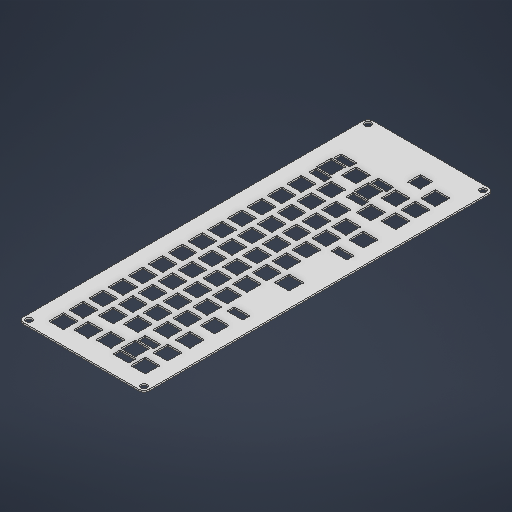
# Autodesk Inventor part: Top_Plate_Mkey
Saved by Autodesk Inventor 2026 (Build 300175050, 175E)
## iProperties
Created: 2025-06-24
Part Number: Top_Plate_Mkey
Material: Generic
Document SubType Name: Modeling
Designer: SaiAn
Density: 1 g/cm^3
Appearance: Default
Author: SaiAn
Autodesk Inventor part; units mm, degrees
ref_plane "YZ Plane" through (0, 0, 0) normal (1, 0, 0) x (0, 1, 0)
ref_plane "XZ Plane" through (0, 0, 0) normal (0, 1, 0) x (-1, 0, 0)
ref_plane "XY Plane" through (0, 0, 0) normal (0, 0, 1) x (1, 0, 0)
sketch "Sketch1" plane through (0, 0, 0) normal (0, 1, 0) x (-1, 0, 0)
  line L0 (0, 0) -> (120.47, 0)
  line L1 (120.47, 0) -> (120.47, -335.78)
  line L2 (120.47, -335.78) -> (0, -335.78)
  line L3 (104.715, -13.9387) -> (104.715, -26.9387)
  line L4 (90.715, -13.9387) -> (90.715, -26.9387)
  line L5 (104.215, -13.4387) -> (91.215, -13.4387)
  line L6 (104.215, -27.4387) -> (91.215, -27.4387)
  arc A0 (104.715, -13.9387) -> (104.215, -13.4387) centre (104.215, -13.9387) ccw
  arc A1 (104.215, -27.4387) -> (104.715, -26.9387) centre (104.215, -26.9387) ccw
  arc A2 (91.215, -13.4387) -> (90.715, -13.9387) centre (91.215, -13.9387) ccw
  arc A3 (90.715, -26.9387) -> (91.215, -27.4387) centre (91.215, -26.9387) ccw
  line L7 (104.715, -32.9887) -> (104.715, -45.9887)
  line L8 (90.715, -32.9887) -> (90.715, -45.9887)
  line L9 (104.215, -32.4887) -> (91.215, -32.4887)
  line L10 (104.215, -46.4887) -> (91.215, -46.4887)
  arc A4 (104.715, -32.9887) -> (104.215, -32.4887) centre (104.215, -32.9887) ccw
  arc A5 (104.215, -46.4887) -> (104.715, -45.9887) centre (104.215, -45.9887) ccw
  arc A6 (91.215, -32.4887) -> (90.715, -32.9887) centre (91.215, -32.9887) ccw
  arc A7 (90.715, -45.9887) -> (91.215, -46.4887) centre (91.215, -45.9887) ccw
  line L11 (104.715, -52.0387) -> (104.715, -65.0387)
  line L12 (90.715, -52.0387) -> (90.715, -65.0387)
  line L13 (104.215, -51.5387) -> (91.215, -51.5387)
  line L14 (104.215, -65.5387) -> (91.215, -65.5387)
  arc A8 (104.715, -52.0387) -> (104.215, -51.5387) centre (104.215, -52.0387) ccw
  arc A9 (104.215, -65.5387) -> (104.715, -65.0387) centre (104.215, -65.0387) ccw
  arc A10 (91.215, -51.5387) -> (90.715, -52.0387) centre (91.215, -52.0387) ccw
  arc A11 (90.715, -65.0387) -> (91.215, -65.5387) centre (91.215, -65.0387) ccw
  line L15 (104.715, -71.0887) -> (104.715, -84.0887)
  line L16 (90.715, -71.0887) -> (90.715, -84.0887)
  line L17 (104.215, -70.5887) -> (91.215, -70.5887)
  line L18 (104.215, -84.5887) -> (91.215, -84.5887)
  arc A12 (104.715, -71.0887) -> (104.215, -70.5887) centre (104.215, -71.0887) ccw
  arc A13 (104.215, -84.5887) -> (104.715, -84.0887) centre (104.215, -84.0887) ccw
  arc A14 (91.215, -70.5887) -> (90.715, -71.0887) centre (91.215, -71.0887) ccw
  arc A15 (90.715, -84.0887) -> (91.215, -84.5887) centre (91.215, -84.0887) ccw
  line L19 (104.715, -90.1387) -> (104.715, -103.1387)
  line L20 (90.715, -90.1387) -> (90.715, -103.1387)
  line L21 (104.215, -89.6387) -> (91.215, -89.6387)
  line L22 (104.215, -103.6387) -> (91.215, -103.6387)
  arc A16 (104.715, -90.1387) -> (104.215, -89.6387) centre (104.215, -90.1387) ccw
  arc A17 (104.215, -103.6387) -> (104.715, -103.1387) centre (104.215, -103.1387) ccw
  arc A18 (91.215, -89.6387) -> (90.715, -90.1387) centre (91.215, -90.1387) ccw
  arc A19 (90.715, -103.1387) -> (91.215, -103.6387) centre (91.215, -103.1387) ccw
  line L23 (104.715, -109.1887) -> (104.715, -122.1887)
  line L24 (90.715, -109.1887) -> (90.715, -122.1887)
  line L25 (104.215, -108.6887) -> (91.215, -108.6887)
  line L26 (104.215, -122.6887) -> (91.215, -122.6887)
  arc A20 (104.715, -109.1887) -> (104.215, -108.6887) centre (104.215, -109.1887) ccw
  arc A21 (104.215, -122.6887) -> (104.715, -122.1887) centre (104.215, -122.1887) ccw
  arc A22 (91.215, -108.6887) -> (90.715, -109.1887) centre (91.215, -109.1887) ccw
  arc A23 (90.715, -122.1887) -> (91.215, -122.6887) centre (91.215, -122.1887) ccw
  line L27 (104.715, -128.2387) -> (104.715, -141.2387)
  line L28 (90.715, -128.2387) -> (90.715, -141.2387)
  line L29 (104.215, -127.7387) -> (91.215, -127.7387)
  line L30 (104.215, -141.7387) -> (91.215, -141.7387)
  arc A24 (104.715, -128.2387) -> (104.215, -127.7387) centre (104.215, -128.2387) ccw
  arc A25 (104.215, -141.7387) -> (104.715, -141.2387) centre (104.215, -141.2387) ccw
  arc A26 (91.215, -127.7387) -> (90.715, -128.2387) centre (91.215, -128.2387) ccw
  arc A27 (90.715, -141.2387) -> (91.215, -141.7387) centre (91.215, -141.2387) ccw
  line L31 (104.715, -147.2887) -> (104.715, -160.2887)
  line L32 (90.715, -147.2887) -> (90.715, -160.2887)
  line L33 (104.215, -146.7887) -> (91.215, -146.7887)
  line L34 (104.215, -160.7887) -> (91.215, -160.7887)
  arc A28 (104.715, -147.2887) -> (104.215, -146.7887) centre (104.215, -147.2887) ccw
  arc A29 (104.215, -160.7887) -> (104.715, -160.2887) centre (104.215, -160.2887) ccw
  arc A30 (91.215, -146.7887) -> (90.715, -147.2887) centre (91.215, -147.2887) ccw
  arc A31 (90.715, -160.2887) -> (91.215, -160.7887) centre (91.215, -160.2887) ccw
  line L35 (104.715, -166.3387) -> (104.715, -179.3387)
  line L36 (90.715, -166.3387) -> (90.715, -179.3387)
  line L37 (104.215, -165.8387) -> (91.215, -165.8387)
  line L38 (104.215, -179.8387) -> (91.215, -179.8387)
  arc A32 (104.715, -166.3387) -> (104.215, -165.8387) centre (104.215, -166.3387) ccw
  arc A33 (104.215, -179.8387) -> (104.715, -179.3387) centre (104.215, -179.3387) ccw
  arc A34 (91.215, -165.8387) -> (90.715, -166.3387) centre (91.215, -166.3387) ccw
  arc A35 (90.715, -179.3387) -> (91.215, -179.8387) centre (91.215, -179.3387) ccw
  line L39 (104.715, -185.3887) -> (104.715, -198.3887)
  line L40 (90.715, -185.3887) -> (90.715, -198.3887)
  line L41 (104.215, -184.8887) -> (91.215, -184.8887)
  line L42 (104.215, -198.8887) -> (91.215, -198.8887)
  arc A36 (104.715, -185.3887) -> (104.215, -184.8887) centre (104.215, -185.3887) ccw
  arc A37 (104.215, -198.8887) -> (104.715, -198.3887) centre (104.215, -198.3887) ccw
  arc A38 (91.215, -184.8887) -> (90.715, -185.3887) centre (91.215, -185.3887) ccw
  arc A39 (90.715, -198.3887) -> (91.215, -198.8887) centre (91.215, -198.3887) ccw
  line L43 (104.715, -204.4387) -> (104.715, -217.4387)
  line L44 (90.715, -204.4387) -> (90.715, -217.4387)
  line L45 (104.215, -203.9387) -> (91.215, -203.9387)
  line L46 (104.215, -217.9387) -> (91.215, -217.9387)
  arc A40 (104.715, -204.4387) -> (104.215, -203.9387) centre (104.215, -204.4387) ccw
  arc A41 (104.215, -217.9387) -> (104.715, -217.4387) centre (104.215, -217.4387) ccw
  arc A42 (91.215, -203.9387) -> (90.715, -204.4387) centre (91.215, -204.4387) ccw
  arc A43 (90.715, -217.4387) -> (91.215, -217.9387) centre (91.215, -217.4387) ccw
  line L47 (104.715, -223.4887) -> (104.715, -236.4887)
  line L48 (90.715, -223.4887) -> (90.715, -236.4887)
  line L49 (104.215, -222.9887) -> (91.215, -222.9887)
  line L50 (104.215, -236.9887) -> (91.215, -236.9887)
  arc A44 (104.715, -223.4887) -> (104.215, -222.9887) centre (104.215, -223.4887) ccw
  arc A45 (104.215, -236.9887) -> (104.715, -236.4887) centre (104.215, -236.4887) ccw
  arc A46 (91.215, -222.9887) -> (90.715, -223.4887) centre (91.215, -223.4887) ccw
  arc A47 (90.715, -236.4887) -> (91.215, -236.9887) centre (91.215, -236.4887) ccw
  line L51 (104.715, -242.5387) -> (104.715, -255.5387)
  line L52 (90.715, -242.5387) -> (90.715, -255.5387)
  line L53 (104.215, -242.0387) -> (91.215, -242.0387)
  line L54 (104.215, -256.0387) -> (91.215, -256.0387)
  arc A48 (104.715, -242.5387) -> (104.215, -242.0387) centre (104.215, -242.5387) ccw
  arc A49 (104.215, -256.0387) -> (104.715, -255.5387) centre (104.215, -255.5387) ccw
  arc A50 (91.215, -242.0387) -> (90.715, -242.5387) centre (91.215, -242.5387) ccw
  arc A51 (90.715, -255.5387) -> (91.215, -256.0387) centre (91.215, -255.5387) ccw
  line L55 (104.715, -271.1137) -> (104.715, -284.1137)
  line L56 (90.715, -271.1137) -> (90.715, -284.1137)
  line L57 (104.215, -270.6137) -> (91.215, -270.6137)
  line L58 (104.215, -284.6137) -> (91.215, -284.6137)
  arc A52 (104.715, -271.1137) -> (104.215, -270.6137) centre (104.215, -271.1137) ccw
  arc A53 (104.215, -284.6137) -> (104.715, -284.1137) centre (104.215, -284.1137) ccw
  arc A54 (91.215, -270.6137) -> (90.715, -271.1137) centre (91.215, -271.1137) ccw
  arc A55 (90.715, -284.1137) -> (91.215, -284.6137) centre (91.215, -284.1137) ccw
  line L59 (103.715, -262.6757) -> (103.715, -268.6757)
  line L60 (88.715, -262.6757) -> (88.715, -268.6757)
  line L61 (103.215, -262.1757) -> (89.215, -262.1757)
  line L62 (103.215, -269.1757) -> (89.215, -269.1757)
  arc A56 (103.715, -262.6757) -> (103.215, -262.1757) centre (103.215, -262.6757) ccw
  arc A57 (103.215, -269.1757) -> (103.715, -268.6757) centre (103.215, -268.6757) ccw
  arc A58 (89.215, -262.1757) -> (88.715, -262.6757) centre (89.215, -262.6757) ccw
  arc A59 (88.715, -268.6757) -> (89.215, -269.1757) centre (89.215, -268.6757) ccw
  line L63 (103.715, -286.5517) -> (103.715, -292.5517)
  line L64 (88.715, -286.5517) -> (88.715, -292.5517)
  line L65 (103.215, -286.0517) -> (89.215, -286.0517)
  line L66 (103.215, -293.0517) -> (89.215, -293.0517)
  arc A60 (103.715, -286.5517) -> (103.215, -286.0517) centre (103.215, -286.5517) ccw
  arc A61 (103.215, -293.0517) -> (103.715, -292.5517) centre (103.215, -292.5517) ccw
  arc A62 (89.215, -286.0517) -> (88.715, -286.5517) centre (89.215, -286.5517) ccw
  arc A63 (88.715, -292.5517) -> (89.215, -293.0517) centre (89.215, -292.5517) ccw
  line L67 (85.665, -18.7012) -> (85.665, -31.7012)
  line L68 (71.665, -18.7012) -> (71.665, -31.7012)
  line L69 (85.165, -18.2012) -> (72.165, -18.2012)
  line L70 (85.165, -32.2012) -> (72.165, -32.2012)
  arc A64 (85.665, -18.7012) -> (85.165, -18.2012) centre (85.165, -18.7012) ccw
  arc A65 (85.165, -32.2012) -> (85.665, -31.7012) centre (85.165, -31.7012) ccw
  arc A66 (72.165, -18.2012) -> (71.665, -18.7012) centre (72.165, -18.7012) ccw
  arc A67 (71.665, -31.7012) -> (72.165, -32.2012) centre (72.165, -31.7012) ccw
  line L71 (85.665, -42.5137) -> (85.665, -55.5137)
  line L72 (71.665, -42.5137) -> (71.665, -55.5137)
  line L73 (85.165, -42.0137) -> (72.165, -42.0137)
  line L74 (85.165, -56.0137) -> (72.165, -56.0137)
  arc A68 (85.665, -42.5137) -> (85.165, -42.0137) centre (85.165, -42.5137) ccw
  arc A69 (85.165, -56.0137) -> (85.665, -55.5137) centre (85.165, -55.5137) ccw
  arc A70 (72.165, -42.0137) -> (71.665, -42.5137) centre (72.165, -42.5137) ccw
  arc A71 (71.665, -55.5137) -> (72.165, -56.0137) centre (72.165, -55.5137) ccw
  line L75 (85.665, -61.5637) -> (85.665, -74.5637)
  line L76 (71.665, -61.5637) -> (71.665, -74.5637)
  line L77 (85.165, -61.0637) -> (72.165, -61.0637)
  line L78 (85.165, -75.0637) -> (72.165, -75.0637)
  arc A72 (85.665, -61.5637) -> (85.165, -61.0637) centre (85.165, -61.5637) ccw
  arc A73 (85.165, -75.0637) -> (85.665, -74.5637) centre (85.165, -74.5637) ccw
  arc A74 (72.165, -61.0637) -> (71.665, -61.5637) centre (72.165, -61.5637) ccw
  arc A75 (71.665, -74.5637) -> (72.165, -75.0637) centre (72.165, -74.5637) ccw
  line L79 (85.665, -80.6137) -> (85.665, -93.6137)
  line L80 (71.665, -80.6137) -> (71.665, -93.6137)
  line L81 (85.165, -80.1137) -> (72.165, -80.1137)
  line L82 (85.165, -94.1137) -> (72.165, -94.1137)
  arc A76 (85.665, -80.6137) -> (85.165, -80.1137) centre (85.165, -80.6137) ccw
  arc A77 (85.165, -94.1137) -> (85.665, -93.6137) centre (85.165, -93.6137) ccw
  arc A78 (72.165, -80.1137) -> (71.665, -80.6137) centre (72.165, -80.6137) ccw
  arc A79 (71.665, -93.6137) -> (72.165, -94.1137) centre (72.165, -93.6137) ccw
  line L83 (85.665, -99.6637) -> (85.665, -112.6637)
  line L84 (71.665, -99.6637) -> (71.665, -112.6637)
  line L85 (85.165, -99.1637) -> (72.165, -99.1637)
  line L86 (85.165, -113.1637) -> (72.165, -113.1637)
  arc A80 (85.665, -99.6637) -> (85.165, -99.1637) centre (85.165, -99.6637) ccw
  arc A81 (85.165, -113.1637) -> (85.665, -112.6637) centre (85.165, -112.6637) ccw
  arc A82 (72.165, -99.1637) -> (71.665, -99.6637) centre (72.165, -99.6637) ccw
  arc A83 (71.665, -112.6637) -> (72.165, -113.1637) centre (72.165, -112.6637) ccw
  line L87 (85.665, -118.7137) -> (85.665, -131.7137)
  line L88 (71.665, -118.7137) -> (71.665, -131.7137)
  line L89 (85.165, -118.2137) -> (72.165, -118.2137)
  line L90 (85.165, -132.2137) -> (72.165, -132.2137)
  arc A84 (85.665, -118.7137) -> (85.165, -118.2137) centre (85.165, -118.7137) ccw
  arc A85 (85.165, -132.2137) -> (85.665, -131.7137) centre (85.165, -131.7137) ccw
  arc A86 (72.165, -118.2137) -> (71.665, -118.7137) centre (72.165, -118.7137) ccw
  arc A87 (71.665, -131.7137) -> (72.165, -132.2137) centre (72.165, -131.7137) ccw
  line L91 (85.665, -137.7637) -> (85.665, -150.7637)
  line L92 (71.665, -137.7637) -> (71.665, -150.7637)
  line L93 (85.165, -137.2637) -> (72.165, -137.2637)
  line L94 (85.165, -151.2637) -> (72.165, -151.2637)
  arc A88 (85.665, -137.7637) -> (85.165, -137.2637) centre (85.165, -137.7637) ccw
  arc A89 (85.165, -151.2637) -> (85.665, -150.7637) centre (85.165, -150.7637) ccw
  arc A90 (72.165, -137.2637) -> (71.665, -137.7637) centre (72.165, -137.7637) ccw
  arc A91 (71.665, -150.7637) -> (72.165, -151.2637) centre (72.165, -150.7637) ccw
  line L95 (85.665, -156.8137) -> (85.665, -169.8137)
  line L96 (71.665, -156.8137) -> (71.665, -169.8137)
  line L97 (85.165, -156.3137) -> (72.165, -156.3137)
  line L98 (85.165, -170.3137) -> (72.165, -170.3137)
  arc A92 (85.665, -156.8137) -> (85.165, -156.3137) centre (85.165, -156.8137) ccw
  arc A93 (85.165, -170.3137) -> (85.665, -169.8137) centre (85.165, -169.8137) ccw
  arc A94 (72.165, -156.3137) -> (71.665, -156.8137) centre (72.165, -156.8137) ccw
  arc A95 (71.665, -169.8137) -> (72.165, -170.3137) centre (72.165, -169.8137) ccw
  line L99 (85.665, -175.8637) -> (85.665, -188.8637)
  line L100 (71.665, -175.8637) -> (71.665, -188.8637)
  line L101 (85.165, -175.3637) -> (72.165, -175.3637)
  line L102 (85.165, -189.3637) -> (72.165, -189.3637)
  arc A96 (85.665, -175.8637) -> (85.165, -175.3637) centre (85.165, -175.8637) ccw
  arc A97 (85.165, -189.3637) -> (85.665, -188.8637) centre (85.165, -188.8637) ccw
  arc A98 (72.165, -175.3637) -> (71.665, -175.8637) centre (72.165, -175.8637) ccw
  arc A99 (71.665, -188.8637) -> (72.165, -189.3637) centre (72.165, -188.8637) ccw
  line L103 (85.665, -194.9137) -> (85.665, -207.9137)
  line L104 (71.665, -194.9137) -> (71.665, -207.9137)
  line L105 (85.165, -194.4137) -> (72.165, -194.4137)
  line L106 (85.165, -208.4137) -> (72.165, -208.4137)
  arc A100 (85.665, -194.9137) -> (85.165, -194.4137) centre (85.165, -194.9137) ccw
  arc A101 (85.165, -208.4137) -> (85.665, -207.9137) centre (85.165, -207.9137) ccw
  arc A102 (72.165, -194.4137) -> (71.665, -194.9137) centre (72.165, -194.9137) ccw
  arc A103 (71.665, -207.9137) -> (72.165, -208.4137) centre (72.165, -207.9137) ccw
  line L107 (85.665, -213.9637) -> (85.665, -226.9637)
  line L108 (71.665, -213.9637) -> (71.665, -226.9637)
  line L109 (85.165, -213.4637) -> (72.165, -213.4637)
  line L110 (85.165, -227.4637) -> (72.165, -227.4637)
  arc A104 (85.665, -213.9637) -> (85.165, -213.4637) centre (85.165, -213.9637) ccw
  arc A105 (85.165, -227.4637) -> (85.665, -226.9637) centre (85.165, -226.9637) ccw
  arc A106 (72.165, -213.4637) -> (71.665, -213.9637) centre (72.165, -213.9637) ccw
  arc A107 (71.665, -226.9637) -> (72.165, -227.4637) centre (72.165, -226.9637) ccw
  line L111 (85.665, -233.0137) -> (85.665, -246.0137)
  line L112 (71.665, -233.0137) -> (71.665, -246.0137)
  line L113 (85.165, -232.5137) -> (72.165, -232.5137)
  line L114 (85.165, -246.5137) -> (72.165, -246.5137)
  arc A108 (85.665, -233.0137) -> (85.165, -232.5137) centre (85.165, -233.0137) ccw
  arc A109 (85.165, -246.5137) -> (85.665, -246.0137) centre (85.165, -246.0137) ccw
  arc A110 (72.165, -232.5137) -> (71.665, -233.0137) centre (72.165, -233.0137) ccw
  arc A111 (71.665, -246.0137) -> (72.165, -246.5137) centre (72.165, -246.0137) ccw
  line L115 (85.665, -252.0637) -> (85.665, -265.0637)
  line L116 (71.665, -252.0637) -> (71.665, -265.0637)
  line L117 (85.165, -251.5637) -> (72.165, -251.5637)
  line L118 (85.165, -265.5637) -> (72.165, -265.5637)
  arc A112 (85.665, -252.0637) -> (85.165, -251.5637) centre (85.165, -252.0637) ccw
  arc A113 (85.165, -265.5637) -> (85.665, -265.0637) centre (85.165, -265.0637) ccw
  arc A114 (72.165, -251.5637) -> (71.665, -252.0637) centre (72.165, -252.0637) ccw
  arc A115 (71.665, -265.0637) -> (72.165, -265.5637) centre (72.165, -265.0637) ccw
  line L119 (85.665, -275.8762) -> (85.665, -288.8762)
  line L120 (71.665, -275.8762) -> (71.665, -288.8762)
  line L121 (85.165, -275.3762) -> (72.165, -275.3762)
  line L122 (85.165, -289.3762) -> (72.165, -289.3762)
  arc A116 (85.665, -275.8762) -> (85.165, -275.3762) centre (85.165, -275.8762) ccw
  arc A117 (85.165, -289.3762) -> (85.665, -288.8762) centre (85.165, -288.8762) ccw
  arc A118 (72.165, -275.3762) -> (71.665, -275.8762) centre (72.165, -275.8762) ccw
  arc A119 (71.665, -288.8762) -> (72.165, -289.3762) centre (72.165, -288.8762) ccw
  line L123 (66.615, -21.0825) -> (66.615, -34.0825)
  line L124 (52.615, -21.0825) -> (52.615, -34.0825)
  line L125 (66.115, -20.5825) -> (53.115, -20.5825)
  line L126 (66.115, -34.5825) -> (53.115, -34.5825)
  arc A120 (66.615, -21.0825) -> (66.115, -20.5825) centre (66.115, -21.0825) ccw
  arc A121 (66.115, -34.5825) -> (66.615, -34.0825) centre (66.115, -34.0825) ccw
  arc A122 (53.115, -20.5825) -> (52.615, -21.0825) centre (53.115, -21.0825) ccw
  arc A123 (52.615, -34.0825) -> (53.115, -34.5825) centre (53.115, -34.0825) ccw
  line L127 (66.615, -47.2762) -> (66.615, -60.2762)
  line L128 (52.615, -47.2762) -> (52.615, -60.2762)
  line L129 (66.115, -46.7762) -> (53.115, -46.7762)
  line L130 (66.115, -60.7762) -> (53.115, -60.7762)
  arc A124 (66.615, -47.2762) -> (66.115, -46.7762) centre (66.115, -47.2762) ccw
  arc A125 (66.115, -60.7762) -> (66.615, -60.2762) centre (66.115, -60.2762) ccw
  arc A126 (53.115, -46.7762) -> (52.615, -47.2762) centre (53.115, -47.2762) ccw
  arc A127 (52.615, -60.2762) -> (53.115, -60.7762) centre (53.115, -60.2762) ccw
  line L131 (66.615, -66.3262) -> (66.615, -79.3262)
  line L132 (52.615, -66.3262) -> (52.615, -79.3262)
  line L133 (66.115, -65.8262) -> (53.115, -65.8262)
  line L134 (66.115, -79.8262) -> (53.115, -79.8262)
  arc A128 (66.615, -66.3262) -> (66.115, -65.8262) centre (66.115, -66.3262) ccw
  arc A129 (66.115, -79.8262) -> (66.615, -79.3262) centre (66.115, -79.3262) ccw
  arc A130 (53.115, -65.8262) -> (52.615, -66.3262) centre (53.115, -66.3262) ccw
  arc A131 (52.615, -79.3262) -> (53.115, -79.8262) centre (53.115, -79.3262) ccw
  line L135 (66.615, -85.3762) -> (66.615, -98.3762)
  line L136 (52.615, -85.3762) -> (52.615, -98.3762)
  line L137 (66.115, -84.8762) -> (53.115, -84.8762)
  line L138 (66.115, -98.8762) -> (53.115, -98.8762)
  arc A132 (66.615, -85.3762) -> (66.115, -84.8762) centre (66.115, -85.3762) ccw
  arc A133 (66.115, -98.8762) -> (66.615, -98.3762) centre (66.115, -98.3762) ccw
  arc A134 (53.115, -84.8762) -> (52.615, -85.3762) centre (53.115, -85.3762) ccw
  arc A135 (52.615, -98.3762) -> (53.115, -98.8762) centre (53.115, -98.3762) ccw
  line L139 (66.615, -104.4262) -> (66.615, -117.4262)
  line L140 (52.615, -104.4262) -> (52.615, -117.4262)
  line L141 (66.115, -103.9262) -> (53.115, -103.9262)
  line L142 (66.115, -117.9262) -> (53.115, -117.9262)
  arc A136 (66.615, -104.4262) -> (66.115, -103.9262) centre (66.115, -104.4262) ccw
  arc A137 (66.115, -117.9262) -> (66.615, -117.4262) centre (66.115, -117.4262) ccw
  arc A138 (53.115, -103.9262) -> (52.615, -104.4262) centre (53.115, -104.4262) ccw
  arc A139 (52.615, -117.4262) -> (53.115, -117.9262) centre (53.115, -117.4262) ccw
  line L143 (66.615, -123.4762) -> (66.615, -136.4762)
  line L144 (52.615, -123.4762) -> (52.615, -136.4762)
  line L145 (66.115, -122.9762) -> (53.115, -122.9762)
  line L146 (66.115, -136.9762) -> (53.115, -136.9762)
  arc A140 (66.615, -123.4762) -> (66.115, -122.9762) centre (66.115, -123.4762) ccw
  arc A141 (66.115, -136.9762) -> (66.615, -136.4762) centre (66.115, -136.4762) ccw
  arc A142 (53.115, -122.9762) -> (52.615, -123.4762) centre (53.115, -123.4762) ccw
  arc A143 (52.615, -136.4762) -> (53.115, -136.9762) centre (53.115, -136.4762) ccw
  line L147 (66.615, -142.5262) -> (66.615, -155.5262)
  line L148 (52.615, -142.5262) -> (52.615, -155.5262)
  line L149 (66.115, -142.0262) -> (53.115, -142.0262)
  line L150 (66.115, -156.0262) -> (53.115, -156.0262)
  arc A144 (66.615, -142.5262) -> (66.115, -142.0262) centre (66.115, -142.5262) ccw
  arc A145 (66.115, -156.0262) -> (66.615, -155.5262) centre (66.115, -155.5262) ccw
  arc A146 (53.115, -142.0262) -> (52.615, -142.5262) centre (53.115, -142.5262) ccw
  arc A147 (52.615, -155.5262) -> (53.115, -156.0262) centre (53.115, -155.5262) ccw
  line L151 (66.615, -161.5762) -> (66.615, -174.5762)
  line L152 (52.615, -161.5762) -> (52.615, -174.5762)
  line L153 (66.115, -161.0762) -> (53.115, -161.0762)
  line L154 (66.115, -175.0762) -> (53.115, -175.0762)
  arc A148 (66.615, -161.5762) -> (66.115, -161.0762) centre (66.115, -161.5762) ccw
  arc A149 (66.115, -175.0762) -> (66.615, -174.5762) centre (66.115, -174.5762) ccw
  arc A150 (53.115, -161.0762) -> (52.615, -161.5762) centre (53.115, -161.5762) ccw
  arc A151 (52.615, -174.5762) -> (53.115, -175.0762) centre (53.115, -174.5762) ccw
  line L155 (66.615, -180.6262) -> (66.615, -193.6262)
  line L156 (52.615, -180.6262) -> (52.615, -193.6262)
  line L157 (66.115, -180.1262) -> (53.115, -180.1262)
  line L158 (66.115, -194.1262) -> (53.115, -194.1262)
  arc A152 (66.615, -180.6262) -> (66.115, -180.1262) centre (66.115, -180.6262) ccw
  arc A153 (66.115, -194.1262) -> (66.615, -193.6262) centre (66.115, -193.6262) ccw
  arc A154 (53.115, -180.1262) -> (52.615, -180.6262) centre (53.115, -180.6262) ccw
  arc A155 (52.615, -193.6262) -> (53.115, -194.1262) centre (53.115, -193.6262) ccw
  line L159 (66.615, -199.6762) -> (66.615, -212.6762)
  line L160 (52.615, -199.6762) -> (52.615, -212.6762)
  line L161 (66.115, -199.1762) -> (53.115, -199.1762)
  line L162 (66.115, -213.1762) -> (53.115, -213.1762)
  arc A156 (66.615, -199.6762) -> (66.115, -199.1762) centre (66.115, -199.6762) ccw
  arc A157 (66.115, -213.1762) -> (66.615, -212.6762) centre (66.115, -212.6762) ccw
  arc A158 (53.115, -199.1762) -> (52.615, -199.6762) centre (53.115, -199.6762) ccw
  arc A159 (52.615, -212.6762) -> (53.115, -213.1762) centre (53.115, -212.6762) ccw
  line L163 (66.615, -218.7262) -> (66.615, -231.7262)
  line L164 (52.615, -218.7262) -> (52.615, -231.7262)
  line L165 (66.115, -218.2262) -> (53.115, -218.2262)
  line L166 (66.115, -232.2262) -> (53.115, -232.2262)
  arc A160 (66.615, -218.7262) -> (66.115, -218.2262) centre (66.115, -218.7262) ccw
  arc A161 (66.115, -232.2262) -> (66.615, -231.7262) centre (66.115, -231.7262) ccw
  arc A162 (53.115, -218.2262) -> (52.615, -218.7262) centre (53.115, -218.7262) ccw
  arc A163 (52.615, -231.7262) -> (53.115, -232.2262) centre (53.115, -231.7262) ccw
  line L167 (66.615, -237.7762) -> (66.615, -250.7762)
  line L168 (52.615, -237.7762) -> (52.615, -250.7762)
  line L169 (66.115, -237.2762) -> (53.115, -237.2762)
  line L170 (66.115, -251.2762) -> (53.115, -251.2762)
  arc A164 (66.615, -237.7762) -> (66.115, -237.2762) centre (66.115, -237.7762) ccw
  arc A165 (66.115, -251.2762) -> (66.615, -250.7762) centre (66.115, -250.7762) ccw
  arc A166 (53.115, -237.2762) -> (52.615, -237.7762) centre (53.115, -237.7762) ccw
  arc A167 (52.615, -250.7762) -> (53.115, -251.2762) centre (53.115, -250.7762) ccw
  line L171 (66.615, -268.7325) -> (66.615, -281.7325)
  line L172 (52.615, -268.7325) -> (52.615, -281.7325)
  line L173 (66.115, -268.2325) -> (53.115, -268.2325)
  line L174 (66.115, -282.2325) -> (53.115, -282.2325)
  arc A168 (66.615, -268.7325) -> (66.115, -268.2325) centre (66.115, -268.7325) ccw
  arc A169 (66.115, -282.2325) -> (66.615, -281.7325) centre (66.115, -281.7325) ccw
  arc A170 (53.115, -268.2325) -> (52.615, -268.7325) centre (53.115, -268.7325) ccw
  arc A171 (52.615, -281.7325) -> (53.115, -282.2325) centre (53.115, -281.7325) ccw
  line L175 (65.615, -260.2945) -> (65.615, -266.2945)
  line L176 (50.615, -260.2945) -> (50.615, -266.2945)
  line L177 (65.115, -259.7945) -> (51.115, -259.7945)
  line L178 (65.115, -266.7945) -> (51.115, -266.7945)
  arc A172 (65.615, -260.2945) -> (65.115, -259.7945) centre (65.115, -260.2945) ccw
  arc A173 (65.115, -266.7945) -> (65.615, -266.2945) centre (65.115, -266.2945) ccw
  arc A174 (51.115, -259.7945) -> (50.615, -260.2945) centre (51.115, -260.2945) ccw
  arc A175 (50.615, -266.2945) -> (51.115, -266.7945) centre (51.115, -266.2945) ccw
  line L179 (65.615, -284.1705) -> (65.615, -290.1705)
  line L180 (50.615, -284.1705) -> (50.615, -290.1705)
  line L181 (65.115, -283.6705) -> (51.115, -283.6705)
  line L182 (65.115, -290.6705) -> (51.115, -290.6705)
  arc A176 (65.615, -284.1705) -> (65.115, -283.6705) centre (65.115, -284.1705) ccw
  arc A177 (65.115, -290.6705) -> (65.615, -290.1705) centre (65.115, -290.1705) ccw
  arc A178 (51.115, -283.6705) -> (50.615, -284.1705) centre (51.115, -284.1705) ccw
  arc A179 (50.615, -290.1705) -> (51.115, -290.6705) centre (51.115, -290.1705) ccw
  line L183 (47.565, -25.845) -> (47.565, -38.845)
  line L184 (33.565, -25.845) -> (33.565, -38.845)
  line L185 (47.065, -25.345) -> (34.065, -25.345)
  line L186 (47.065, -39.345) -> (34.065, -39.345)
  arc A180 (47.565, -25.845) -> (47.065, -25.345) centre (47.065, -25.845) ccw
  arc A181 (47.065, -39.345) -> (47.565, -38.845) centre (47.065, -38.845) ccw
  arc A182 (34.065, -25.345) -> (33.565, -25.845) centre (34.065, -25.845) ccw
  arc A183 (33.565, -38.845) -> (34.065, -39.345) centre (34.065, -38.845) ccw
  line L187 (46.565, -17.407) -> (46.565, -23.407)
  line L188 (31.565, -17.407) -> (31.565, -23.407)
  line L189 (46.065, -16.907) -> (32.065, -16.907)
  line L190 (46.065, -23.907) -> (32.065, -23.907)
  arc A184 (46.565, -17.407) -> (46.065, -16.907) centre (46.065, -17.407) ccw
  arc A185 (46.065, -23.907) -> (46.565, -23.407) centre (46.065, -23.407) ccw
  arc A186 (32.065, -16.907) -> (31.565, -17.407) centre (32.065, -17.407) ccw
  arc A187 (31.565, -23.407) -> (32.065, -23.907) centre (32.065, -23.407) ccw
  line L191 (46.565, -41.283) -> (46.565, -47.283)
  line L192 (31.565, -41.283) -> (31.565, -47.283)
  line L193 (46.065, -40.783) -> (32.065, -40.783)
  line L194 (46.065, -47.783) -> (32.065, -47.783)
  arc A188 (46.565, -41.283) -> (46.065, -40.783) centre (46.065, -41.283) ccw
  arc A189 (46.065, -47.783) -> (46.565, -47.283) centre (46.065, -47.283) ccw
  arc A190 (32.065, -40.783) -> (31.565, -41.283) centre (32.065, -41.283) ccw
  arc A191 (31.565, -47.283) -> (32.065, -47.783) centre (32.065, -47.283) ccw
  line L195 (47.565, -56.8012) -> (47.565, -69.8012)
  line L196 (33.565, -56.8012) -> (33.565, -69.8012)
  line L197 (47.065, -56.3012) -> (34.065, -56.3012)
  line L198 (47.065, -70.3012) -> (34.065, -70.3012)
  arc A192 (47.565, -56.8012) -> (47.065, -56.3012) centre (47.065, -56.8012) ccw
  arc A193 (47.065, -70.3012) -> (47.565, -69.8012) centre (47.065, -69.8012) ccw
  arc A194 (34.065, -56.3012) -> (33.565, -56.8012) centre (34.065, -56.8012) ccw
  arc A195 (33.565, -69.8012) -> (34.065, -70.3012) centre (34.065, -69.8012) ccw
  line L199 (47.565, -75.8512) -> (47.565, -88.8512)
  line L200 (33.565, -75.8512) -> (33.565, -88.8512)
  line L201 (47.065, -75.3512) -> (34.065, -75.3512)
  line L202 (47.065, -89.3512) -> (34.065, -89.3512)
  arc A196 (47.565, -75.8512) -> (47.065, -75.3512) centre (47.065, -75.8512) ccw
  arc A197 (47.065, -89.3512) -> (47.565, -88.8512) centre (47.065, -88.8512) ccw
  arc A198 (34.065, -75.3512) -> (33.565, -75.8512) centre (34.065, -75.8512) ccw
  arc A199 (33.565, -88.8512) -> (34.065, -89.3512) centre (34.065, -88.8512) ccw
  line L203 (47.565, -94.9012) -> (47.565, -107.9012)
  line L204 (33.565, -94.9012) -> (33.565, -107.9012)
  line L205 (47.065, -94.4012) -> (34.065, -94.4012)
  line L206 (47.065, -108.4012) -> (34.065, -108.4012)
  arc A200 (47.565, -94.9012) -> (47.065, -94.4012) centre (47.065, -94.9012) ccw
  arc A201 (47.065, -108.4012) -> (47.565, -107.9012) centre (47.065, -107.9012) ccw
  arc A202 (34.065, -94.4012) -> (33.565, -94.9012) centre (34.065, -94.9012) ccw
  arc A203 (33.565, -107.9012) -> (34.065, -108.4012) centre (34.065, -107.9012) ccw
  line L207 (47.565, -113.9512) -> (47.565, -126.9512)
  line L208 (33.565, -113.9512) -> (33.565, -126.9512)
  line L209 (47.065, -113.4512) -> (34.065, -113.4512)
  line L210 (47.065, -127.4512) -> (34.065, -127.4512)
  arc A204 (47.565, -113.9512) -> (47.065, -113.4512) centre (47.065, -113.9512) ccw
  arc A205 (47.065, -127.4512) -> (47.565, -126.9512) centre (47.065, -126.9512) ccw
  arc A206 (34.065, -113.4512) -> (33.565, -113.9512) centre (34.065, -113.9512) ccw
  arc A207 (33.565, -126.9512) -> (34.065, -127.4512) centre (34.065, -126.9512) ccw
  line L211 (47.565, -133.0012) -> (47.565, -146.0012)
  line L212 (33.565, -133.0012) -> (33.565, -146.0012)
  line L213 (47.065, -132.5012) -> (34.065, -132.5012)
  line L214 (47.065, -146.5012) -> (34.065, -146.5012)
  arc A208 (47.565, -133.0012) -> (47.065, -132.5012) centre (47.065, -133.0012) ccw
  arc A209 (47.065, -146.5012) -> (47.565, -146.0012) centre (47.065, -146.0012) ccw
  arc A210 (34.065, -132.5012) -> (33.565, -133.0012) centre (34.065, -133.0012) ccw
  arc A211 (33.565, -146.0012) -> (34.065, -146.5012) centre (34.065, -146.0012) ccw
  line L215 (47.565, -152.0512) -> (47.565, -165.0512)
  line L216 (33.565, -152.0512) -> (33.565, -165.0512)
  line L217 (47.065, -151.5512) -> (34.065, -151.5512)
  line L218 (47.065, -165.5512) -> (34.065, -165.5512)
  arc A212 (47.565, -152.0512) -> (47.065, -151.5512) centre (47.065, -152.0512) ccw
  arc A213 (47.065, -165.5512) -> (47.565, -165.0512) centre (47.065, -165.0512) ccw
  arc A214 (34.065, -151.5512) -> (33.565, -152.0512) centre (34.065, -152.0512) ccw
  arc A215 (33.565, -165.0512) -> (34.065, -165.5512) centre (34.065, -165.0512) ccw
  line L219 (47.565, -171.1012) -> (47.565, -184.1012)
  line L220 (33.565, -171.1012) -> (33.565, -184.1012)
  line L221 (47.065, -170.6012) -> (34.065, -170.6012)
  line L222 (47.065, -184.6012) -> (34.065, -184.6012)
  arc A216 (47.565, -171.1012) -> (47.065, -170.6012) centre (47.065, -171.1012) ccw
  arc A217 (47.065, -184.6012) -> (47.565, -184.1012) centre (47.065, -184.1012) ccw
  arc A218 (34.065, -170.6012) -> (33.565, -171.1012) centre (34.065, -171.1012) ccw
  arc A219 (33.565, -184.1012) -> (34.065, -184.6012) centre (34.065, -184.1012) ccw
  line L223 (47.565, -190.1512) -> (47.565, -203.1512)
  line L224 (33.565, -190.1512) -> (33.565, -203.1512)
  line L225 (47.065, -189.6512) -> (34.065, -189.6512)
  line L226 (47.065, -203.6512) -> (34.065, -203.6512)
  arc A220 (47.565, -190.1512) -> (47.065, -189.6512) centre (47.065, -190.1512) ccw
  arc A221 (47.065, -203.6512) -> (47.565, -203.1512) centre (47.065, -203.1512) ccw
  arc A222 (34.065, -189.6512) -> (33.565, -190.1512) centre (34.065, -190.1512) ccw
  arc A223 (33.565, -203.1512) -> (34.065, -203.6512) centre (34.065, -203.1512) ccw
  line L227 (47.565, -209.2012) -> (47.565, -222.2012)
  line L228 (33.565, -209.2012) -> (33.565, -222.2012)
  line L229 (47.065, -208.7012) -> (34.065, -208.7012)
  line L230 (47.065, -222.7012) -> (34.065, -222.7012)
  arc A224 (47.565, -209.2012) -> (47.065, -208.7012) centre (47.065, -209.2012) ccw
  arc A225 (47.065, -222.7012) -> (47.565, -222.2012) centre (47.065, -222.2012) ccw
  arc A226 (34.065, -208.7012) -> (33.565, -209.2012) centre (34.065, -209.2012) ccw
  arc A227 (33.565, -222.2012) -> (34.065, -222.7012) centre (34.065, -222.2012) ccw
  line L231 (47.565, -228.2512) -> (47.565, -241.2512)
  line L232 (33.565, -228.2512) -> (33.565, -241.2512)
  line L233 (47.065, -227.7512) -> (34.065, -227.7512)
  line L234 (47.065, -241.7512) -> (34.065, -241.7512)
  arc A228 (47.565, -228.2512) -> (47.065, -227.7512) centre (47.065, -228.2512) ccw
  arc A229 (47.065, -241.7512) -> (47.565, -241.2512) centre (47.065, -241.2512) ccw
  arc A230 (34.065, -227.7512) -> (33.565, -228.2512) centre (34.065, -228.2512) ccw
  arc A231 (33.565, -241.2512) -> (34.065, -241.7512) centre (34.065, -241.2512) ccw
  line L235 (47.565, -252.0637) -> (47.565, -265.0637)
  line L236 (33.565, -252.0637) -> (33.565, -265.0637)
  line L237 (47.065, -251.5637) -> (34.065, -251.5637)
  line L238 (47.065, -265.5637) -> (34.065, -265.5637)
  arc A232 (47.565, -252.0637) -> (47.065, -251.5637) centre (47.065, -252.0637) ccw
  arc A233 (47.065, -265.5637) -> (47.565, -265.0637) centre (47.065, -265.0637) ccw
  arc A234 (34.065, -251.5637) -> (33.565, -252.0637) centre (34.065, -252.0637) ccw
  arc A235 (33.565, -265.0637) -> (34.065, -265.5637) centre (34.065, -265.0637) ccw
  line L239 (47.565, -275.8762) -> (47.565, -288.8762)
  line L240 (33.565, -275.8762) -> (33.565, -288.8762)
  line L241 (47.065, -275.3762) -> (34.065, -275.3762)
  line L242 (47.065, -289.3762) -> (34.065, -289.3762)
  arc A236 (47.565, -275.8762) -> (47.065, -275.3762) centre (47.065, -275.8762) ccw
  arc A237 (47.065, -289.3762) -> (47.565, -288.8762) centre (47.065, -288.8762) ccw
  arc A238 (34.065, -275.3762) -> (33.565, -275.8762) centre (34.065, -275.8762) ccw
  arc A239 (33.565, -288.8762) -> (34.065, -289.3762) centre (34.065, -288.8762) ccw
  line L243 (28.515, -16.32) -> (28.515, -29.32)
  line L244 (14.515, -16.32) -> (14.515, -29.32)
  line L245 (28.015, -15.82) -> (15.015, -15.82)
  line L246 (28.015, -29.82) -> (15.015, -29.82)
  arc A240 (28.515, -16.32) -> (28.015, -15.82) centre (28.015, -16.32) ccw
  arc A241 (28.015, -29.82) -> (28.515, -29.32) centre (28.015, -29.32) ccw
  arc A242 (15.015, -15.82) -> (14.515, -16.32) centre (15.015, -16.32) ccw
  arc A243 (14.515, -29.32) -> (15.015, -29.82) centre (15.015, -29.32) ccw
  line L247 (28.515, -37.7512) -> (28.515, -50.7512)
  line L248 (14.515, -37.7512) -> (14.515, -50.7512)
  line L249 (28.015, -37.2512) -> (15.015, -37.2512)
  line L250 (28.015, -51.2512) -> (15.015, -51.2512)
  arc A244 (28.515, -37.7512) -> (28.015, -37.2512) centre (28.015, -37.7512) ccw
  arc A245 (28.015, -51.2512) -> (28.515, -50.7512) centre (28.015, -50.7512) ccw
  arc A246 (15.015, -37.2512) -> (14.515, -37.7512) centre (15.015, -37.7512) ccw
  arc A247 (14.515, -50.7512) -> (15.015, -51.2512) centre (15.015, -50.7512) ccw
  line L251 (28.515, -59.1825) -> (28.515, -72.1825)
  line L252 (14.515, -59.1825) -> (14.515, -72.1825)
  line L253 (28.015, -58.6825) -> (15.015, -58.6825)
  line L254 (28.015, -72.6825) -> (15.015, -72.6825)
  arc A248 (28.515, -59.1825) -> (28.015, -58.6825) centre (28.015, -59.1825) ccw
  arc A249 (28.015, -72.6825) -> (28.515, -72.1825) centre (28.015, -72.1825) ccw
  arc A250 (15.015, -58.6825) -> (14.515, -59.1825) centre (15.015, -59.1825) ccw
  arc A251 (14.515, -72.1825) -> (15.015, -72.6825) centre (15.015, -72.1825) ccw
  line L255 (28.515, -82.995) -> (28.515, -95.995)
  line L256 (14.515, -82.995) -> (14.515, -95.995)
  line L257 (28.015, -82.495) -> (15.015, -82.495)
  line L258 (28.015, -96.495) -> (15.015, -96.495)
  arc A252 (28.515, -82.995) -> (28.015, -82.495) centre (28.015, -82.995) ccw
  arc A253 (28.015, -96.495) -> (28.515, -95.995) centre (28.015, -95.995) ccw
  arc A254 (15.015, -82.495) -> (14.515, -82.995) centre (15.015, -82.995) ccw
  arc A255 (14.515, -95.995) -> (15.015, -96.495) centre (15.015, -95.995) ccw
  line L259 (28.515, -154.4325) -> (28.515, -167.4325)
  line L260 (14.515, -154.4325) -> (14.515, -167.4325)
  line L261 (28.015, -153.9325) -> (15.015, -153.9325)
  line L262 (28.015, -167.9325) -> (15.015, -167.9325)
  arc A256 (28.515, -154.4325) -> (28.015, -153.9325) centre (28.015, -154.4325) ccw
  arc A257 (28.015, -167.9325) -> (28.515, -167.4325) centre (28.015, -167.4325) ccw
  arc A258 (15.015, -153.9325) -> (14.515, -154.4325) centre (15.015, -154.4325) ccw
  arc A259 (14.515, -167.4325) -> (15.015, -167.9325) centre (15.015, -167.4325) ccw
  line L263 (27.515, -107.9325) -> (27.515, -113.9325)
  line L264 (12.515, -107.9325) -> (12.515, -113.9325)
  line L265 (27.015, -107.4325) -> (13.015, -107.4325)
  line L266 (27.015, -114.4325) -> (13.015, -114.4325)
  arc A260 (27.515, -107.9325) -> (27.015, -107.4325) centre (27.015, -107.9325) ccw
  arc A261 (27.015, -114.4325) -> (27.515, -113.9325) centre (27.015, -113.9325) ccw
  arc A262 (13.015, -107.4325) -> (12.515, -107.9325) centre (13.015, -107.9325) ccw
  arc A263 (12.515, -113.9325) -> (13.015, -114.4325) centre (13.015, -113.9325) ccw
  line L267 (27.515, -207.9325) -> (27.515, -213.9325)
  line L268 (12.515, -207.9325) -> (12.515, -213.9325)
  line L269 (27.015, -207.4325) -> (13.015, -207.4325)
  line L270 (27.015, -214.4325) -> (13.015, -214.4325)
  arc A264 (27.515, -207.9325) -> (27.015, -207.4325) centre (27.015, -207.9325) ccw
  arc A265 (27.015, -214.4325) -> (27.515, -213.9325) centre (27.015, -213.9325) ccw
  arc A266 (13.015, -207.4325) -> (12.515, -207.9325) centre (13.015, -207.9325) ccw
  arc A267 (12.515, -213.9325) -> (13.015, -214.4325) centre (13.015, -213.9325) ccw
  line L271 (28.515, -225.87) -> (28.515, -238.87)
  line L272 (14.515, -225.87) -> (14.515, -238.87)
  line L273 (28.015, -225.37) -> (15.015, -225.37)
  line L274 (28.015, -239.37) -> (15.015, -239.37)
  arc A268 (28.515, -225.87) -> (28.015, -225.37) centre (28.015, -225.87) ccw
  arc A269 (28.015, -239.37) -> (28.515, -238.87) centre (28.015, -238.87) ccw
  arc A270 (15.015, -225.37) -> (14.515, -225.87) centre (15.015, -225.87) ccw
  arc A271 (14.515, -238.87) -> (15.015, -239.37) centre (15.015, -238.87) ccw
  line L275 (28.515, -256.8262) -> (28.515, -269.8262)
  line L276 (14.515, -256.8262) -> (14.515, -269.8262)
  line L277 (28.015, -256.3262) -> (15.015, -256.3262)
  line L278 (28.015, -270.3262) -> (15.015, -270.3262)
  arc A272 (28.515, -256.8262) -> (28.015, -256.3262) centre (28.015, -256.8262) ccw
  arc A273 (28.015, -270.3262) -> (28.515, -269.8262) centre (28.015, -269.8262) ccw
  arc A274 (15.015, -256.3262) -> (14.515, -256.8262) centre (15.015, -256.8262) ccw
  arc A275 (14.515, -269.8262) -> (15.015, -270.3262) centre (15.015, -269.8262) ccw
  line L279 (28.515, -275.8762) -> (28.515, -288.8762)
  line L280 (14.515, -275.8762) -> (14.515, -288.8762)
  line L281 (28.015, -275.3762) -> (15.015, -275.3762)
  line L282 (28.015, -289.3762) -> (15.015, -289.3762)
  arc A276 (28.515, -275.8762) -> (28.015, -275.3762) centre (28.015, -275.8762) ccw
  arc A277 (28.015, -289.3762) -> (28.515, -288.8762) centre (28.015, -288.8762) ccw
  arc A278 (15.015, -275.3762) -> (14.515, -275.8762) centre (15.015, -275.8762) ccw
  arc A279 (14.515, -288.8762) -> (15.015, -289.3762) centre (15.015, -288.8762) ccw
  line L283 (28.515, -294.9262) -> (28.515, -307.9262)
  line L284 (14.515, -294.9262) -> (14.515, -307.9262)
  line L285 (28.015, -294.4262) -> (15.015, -294.4262)
  line L286 (28.015, -308.4262) -> (15.015, -308.4262)
  arc A280 (28.515, -294.9262) -> (28.015, -294.4262) centre (28.015, -294.9262) ccw
  arc A281 (28.015, -308.4262) -> (28.515, -307.9262) centre (28.015, -307.9262) ccw
  arc A282 (15.015, -294.4262) -> (14.515, -294.9262) centre (15.015, -294.9262) ccw
  arc A283 (14.515, -307.9262) -> (15.015, -308.4262) centre (15.015, -307.9262) ccw
  line L287 (0, 0) -> (0, -335.78)
  circle A284 centre (115.47, -5) radius 3
  circle A285 centre (5, -5) radius 3
  circle A286 centre (115.47, -330.78) radius 3
  circle A287 centre (5, -330.78) radius 3
  line L288 (36.455, -301.7362) -> (48.255, -301.7362)
  line L289 (48.255, -301.7362) -> (48.255, -313.9362)
  line L290 (48.255, -313.9362) -> (36.455, -313.9362)
  line L291 (36.455, -313.9362) -> (36.455, -301.7362)
  point P0 (28.515, -238.87)
  point P1 (28.015, -239.37)
  point P2 (28.015, -225.37)
  point P3 (27.015, -207.4325)
  point P4 (28.015, -308.4262)
  point P5 (28.015, -294.4262)
  point P6 (28.515, -294.9262)
  point P7 (28.515, -288.8762)
  point P8 (28.015, -289.3762)
  point P9 (15.015, -289.3762)
  point P10 (28.515, -256.8262)
  point P11 (28.515, -269.8262)
  point P12 (28.015, -270.3262)
  point P13 (14.515, -269.8262)
  point P14 (34.065, -265.5637)
  point P15 (34.065, -251.5637)
  point P16 (47.565, -275.8762)
  point P17 (33.565, -275.8762)
  point P18 (51.115, -290.6705)
  point P19 (66.615, -268.7325)
  point P20 (53.115, -282.2325)
  point P21 (52.615, -268.7325)
  point P22 (53.115, -268.2325)
  point P23 (51.115, -266.7945)
  point P24 (47.565, -222.2012)
  point P25 (47.065, -222.7012)
  point P26 (34.065, -222.7012)
  point P27 (34.065, -208.7012)
  point P28 (34.065, -70.3012)
  point P29 (33.565, -69.8012)
  point P30 (47.565, -88.8512)
  point P31 (33.565, -88.8512)
  point P32 (47.065, -94.4012)
  point P33 (53.115, -251.2762)
  point P34 (53.115, -237.2762)
  point P35 (66.615, -218.7262)
  point P36 (66.115, -199.1762)
  point P37 (66.615, -199.6762)
  point P38 (52.615, -34.0825)
  point P39 (52.615, -47.2762)
  point P40 (53.115, -46.7762)
  point P41 (66.615, -66.3262)
  point P42 (52.615, -79.3262)
  point P43 (47.565, -184.1012)
  point P44 (47.065, -184.6012)
  point P45 (47.565, -190.1512)
  point P46 (47.565, -203.1512)
  point P47 (47.065, -203.6512)
  point P48 (34.065, -203.6512)
  point P49 (33.565, -203.1512)
  point P50 (53.115, -194.1262)
  point P51 (52.615, -180.6262)
  point P52 (53.115, -180.1262)
  point P53 (85.665, -275.8762)
  point P54 (72.165, -289.3762)
  point P55 (71.665, -275.8762)
  point P56 (89.215, -293.0517)
  point P57 (71.665, -55.5137)
  point P58 (72.165, -42.0137)
  point P59 (15.015, -167.9325)
  point P60 (14.515, -167.4325)
  point P61 (85.665, -252.0637)
  point P62 (85.165, -265.5637)
  point P63 (71.665, -252.0637)
  point P64 (72.165, -251.5637)
  point P65 (85.165, -227.4637)
  point P66 (72.165, -227.4637)
  point P67 (52.615, -161.5762)
  point P68 (53.115, -161.0762)
  point P69 (66.115, -161.0762)
  point P70 (66.615, -161.5762)
  point P71 (66.615, -142.5262)
  point P72 (66.115, -156.0262)
  point P73 (53.115, -156.0262)
  point P74 (33.565, -126.9512)
  point P75 (52.615, -136.4762)
  point P76 (52.615, -123.4762)
  point P77 (53.115, -122.9762)
  point P78 (85.165, -118.2137)
  point P79 (66.615, -117.4262)
  point P80 (66.115, -117.9262)
  point P81 (85.665, -99.6637)
  point P82 (71.665, -99.6637)
  point P83 (72.165, -94.1137)
  point P84 (71.665, -93.6137)
  point P85 (85.165, -80.1137)
  point P86 (103.715, -262.6757)
  point P87 (91.215, -256.0387)
  point P88 (90.715, -255.5387)
  point P89 (91.215, -242.0387)
  point P90 (85.165, -246.5137)
  point P91 (72.165, -246.5137)
  point P92 (72.165, -232.5137)
  point P93 (104.215, -236.9887)
  point P94 (90.715, -223.4887)
  point P95 (91.215, -222.9887)
  point P96 (104.715, -204.4387)
  point P97 (90.715, -204.4387)
  dimension "d14" = 120.47
  dimension "d15" = 335.78
  dimension "d18" = 6
  dimension "d19" = 6
  dimension "d20" = 6
  dimension "d21" = 6
  dimension "d22" = 5
  dimension "d23" = 5
  dimension "d24" = 5
  dimension "d25" = 5
  dimension "d26" = 5
  dimension "d27" = 5
  dimension "d28" = 5
  dimension "d29" = 5
  dimension "d32" = 11.8
  dimension "d33" = 12.2
  constraints: 584 end point, 568 point on circle, 288 centre point, 3 parallel, 2 horizontal, 2 perpendicular, 1 vertical
  measures "d14" distance of L1.end L2.end
  measures "d15" distance of L0.end L1.end
  measures "d18" diameter of A284
  measures "d19" diameter of A285
  measures "d20" diameter of A286
  measures "d21" diameter of A287
  measures "d22" distance from line of L1 A284.centre
  measures "d23" distance from line of L0 A284.centre
  measures "d24" distance from line of L287 A285.centre
  measures "d25" distance from line of L0 A285.centre
  measures "d26" distance from line of L287 A287.centre
  measures "d27" distance from line of L2 A287.centre
  measures "d28" distance from line of L1 A286.centre
  measures "d29" distance from line of L2 A286.centre
  measures "d32" distance of L289.end L290.end
  measures "d33" distance of L288.end L289.end
extrude "Extrusion1" add sketch "Sketch1" along normal blind 1.5
fillet "Fillet1" radius 5 4 edges at (-120.47, 0.75, 0) (0, 0.75, 0) (0, 0.75, -335.78) (-120.47, 0.75, -335.78)
body "Solid1"
